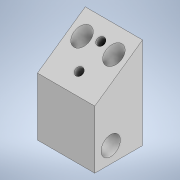
# Autodesk Inventor part: s_base1
Saved by Autodesk Inventor 2022 (Build 260153000, 153)
## iProperties
Created: 2021-08-20
Part Number: s_base1
Material: 一般
Document SubType Name: Modeling
Designer: yuta0
Density: 1 g/cm^3
Appearance: 既定
Author: yuta0
Autodesk Inventor part; units mm, degrees
ref_plane "YZ Plane" through (0, 0, 0) normal (1, 0, 0) x (0, 1, 0)
ref_plane "XZ Plane" through (0, 0, 0) normal (0, 1, 0) x (-1, 0, 0)
ref_plane "XY Plane" through (0, 0, 0) normal (0, 0, 1) x (1, 0, 0)
sketch "スケッチ1" plane through (0, 0, 0) normal (1, 0, 0) x (0, 1, 0)
  line L0 (0, 0) -> (36.4832, 0)
  line L1 (36.4832, 0) -> (57.4894, -30)
  line L2 (57.4894, -30) -> (0, -30)
  line L3 (0, -30) -> (0, 0)
  dimension "d0" = 35
  dimension "d1" = 36.4832
  dimension "d2" = 30
  constraints: 8 end point, 1 horizontal, 1 parallel, 1 perpendicular
  measures "d0" angle of L3 L1
  measures "d1" distance of L0.start L0.end
  measures "d2" distance of L2.end L0.start
extrude "押し出し1" add sketch "スケッチ1" along normal mid plane 36
ref_plane "作業平面1" through (-18, 70, -30) normal (0, -1, 0) x (1, 0, 0)
sketch "スケッチ3" plane through (-18, 70, -30) normal (0, -1, 0) x (1, 0, 0)
  line L0 (0, 0) -> (36, 0) projected
  line L1 (0, 30) -> (0, 0) projected
  line L2 (36, 0) -> (36, 30) projected
  point P0 (18, 30)
  point P1 (8, 10)
  point P2 (28, 10)
  dimension "d11" = 10
  dimension "d12" = 8
  dimension "d13" = 8
  dimension "d14" = 10
  measures "d11" distance from line of L0 point (8, 10)
  measures "d12" distance from line of L1 point (8, 10)
  measures "d13" distance from line of L2 point (28, 10)
  measures "d14" distance from line of L0 point (28, 10)
hole "穴1" at (-10, 70, -20) at (10, 70, -20) direction (0, -1, 0) diameter 5.5 end through all counterbore diameter 10 counterbore depth 30 clearance for "Socket Head Cap Screw" size "M5" standard "Ansi Metric M Profile"
sketch "スケッチ4" plane through (-18, 36.4832, 0) normal (0, 0.819152, 0.5735764) x (1, 0, 0)
  line L0 (18, 10) -> (18, 10)
  line L1 (18, 10) -> (18, 26.6232)
  line L2 (18, 26.6232) -> (18, 26.6232)
  line L3 (18, 26.6232) -> (18, 10)
  line L4 (0, 36.6232) -> (36, 36.6232) projected
  line L5 (0, 0) -> (36, 0) projected
  line L6 (0, 0) -> (0, 36.6232) projected
  line L7 (36, 36.6232) -> (36, 0) projected
  point P0 (18, -20.9259)
  dimension "d22" = 36.6232
  dimension "d24" = 10
  dimension "d36" = 10
  dimension "d46" = 18
  dimension "d47" = 18
  dimension "d51" = 36
  constraints: 8 end point, 2 equal length, 1 horizontal, 1 perpendicular
  measures "d22" distance of L5.end L4.end
  measures "d24" distance between parallel lines of L4 L2
  measures "d36" distance between parallel lines of L5 L0
  measures "d46" distance between parallel lines of L6 L1
  measures "d47" distance between parallel lines of L7 L3
  measures "d51" distance of L4.start L4.end
hole "穴2" at (0, 51.7537, -21.8085) at (0, 42.219, -8.1915) at (0, 51.7537, -21.8085) at (0, 42.219, -8.1915) direction (0, -0.819152, -0.5735764) diameter 5 depth 6 tip angle 118
sketch "スケッチ5" plane through (18, 0, 0) normal (1, 0, 0) x (0, 0, -1)
  circle A0 centre (10, 10) radius 6.05
  line L0 (0, 0) -> (30, 0) projected
  line L1 (0, 36.4832) -> (0, 0) projected
  dimension "d40" = 10
  dimension "d41" = 10
  dimension "d42" = 12.1
  constraints: 1 centre point
  measures "d40" distance from line of L0 A0.centre
  measures "d41" distance from line of L1 A0.centre
  measures "d42" diameter of A0
extrude "押し出し3" cut sketch "スケッチ5" against normal through all
equation "\"d13\" = d12"
equation "\"d14\" = d11"
equation "\"d46\" = 0.5 * d51"
equation "\"d47\" = d46"
